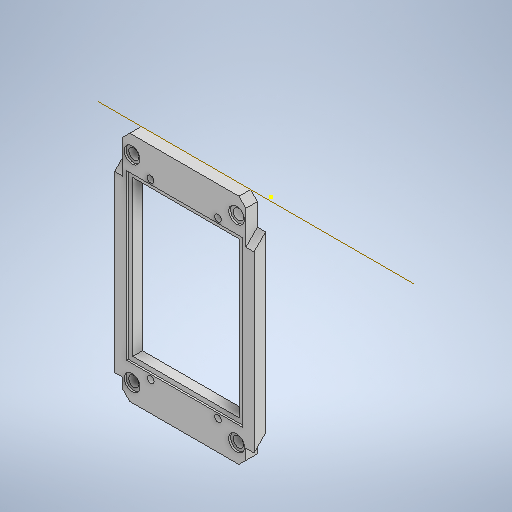
# Autodesk Inventor part: mirror_bracket
Saved by Autodesk Inventor 2025.1 (Build 291241000, 241)
## iProperties
Created: 2024-11-14
Part Number: mirror_bracket
Material: Ogólny
Document SubType Name: Modeling
Designer: PC
Density: 1 g/cm^3
Appearance: Domyślna
Author: PC
Autodesk Inventor part; units mm, degrees
ref_plane "YZ Plane" through (0, 0, 0) normal (1, 0, 0) x (0, 1, 0)
ref_plane "XZ Plane" through (0, 0, 0) normal (0, 1, 0) x (-1, 0, 0)
ref_plane "XY Plane" through (0, 0, 0) normal (0, 0, 1) x (1, 0, 0)
sketch "Szkic1" plane through (0, 0, 0) normal (0, 0, 1) x (1, 0, 0)
  circle A0 centre (-15, -14.1421) radius 2 projected
  circle A1 centre (-60, -14.1421) radius 2 projected
  circle A2 centre (-15, -98.9949) radius 2 projected
  circle A3 centre (-60, -98.9949) radius 2 projected
  line L0 (-75, -84.8528) -> (0, -84.8528) construction
  line L1 (-75, -27.2843) -> (0, -27.2843) construction
  line L2 (-12.5, -21.2132) -> (-62.5, -21.2132) construction
  line L3 (-62.5, -21.2132) -> (-62.5, -91.9239) construction
  line L4 (-62.5, -91.9239) -> (-12.5, -91.9239) construction
  line L5 (-12.5, -91.9239) -> (-12.5, -21.2132) construction
  line L6 (-15, -98.9949) -> (-60, -14.1421) construction
  line L7 (-15, -14.1421) -> (-60, -98.9949) construction
  line L8 (-7.5, -6.5685) -> (-67.5, -6.5685)
  line L9 (-67.5, -6.5685) -> (-67.5, -106.5685)
  line L10 (-67.5, -106.5685) -> (-7.5, -106.5685)
  line L11 (-7.5, -106.5685) -> (-7.5, -6.5685)
  circle A4 centre (-15, -14.1421) radius 2.25
  circle A5 centre (-60, -14.1421) radius 2.25
  circle A6 centre (-60, -98.9949) radius 2.25
  circle A7 centre (-15, -98.9949) radius 2.25
  line L12 (-12.5, -21.2132) -> (-62.5, -21.2132)
  line L13 (-62.5, -21.2132) -> (-62.5, -91.9239)
  line L14 (-62.5, -91.9239) -> (-12.5, -91.9239)
  line L15 (-12.5, -91.9239) -> (-12.5, -21.2132)
  line L16 (-14.5, -23.2132) -> (-60.5, -23.2132)
  line L17 (-60.5, -23.2132) -> (-60.5, -89.9239)
  line L18 (-60.5, -89.9239) -> (-14.5, -89.9239)
  line L19 (-14.5, -89.9239) -> (-14.5, -23.2132)
  ellipse E0 centre (-7.5, -14.1421) end of major axis (-7.5, -18.3848) minor radius 3 projected
  ellipse E1 centre (-67.5, -14.1421) end of major axis (-67.5, -18.3848) minor radius 3 projected
  ellipse E2 centre (-67.5, -98.9949) end of major axis (-67.5, -103.2376) minor radius 3 projected
  ellipse E3 centre (-7.5, -98.9949) end of major axis (-7.5, -103.2376) minor radius 3 projected
  line L20 (-11.5, -94.4949) -> (-11.5, -106.5685)
  line L21 (-11.5, -94.4949) -> (-7.5, -94.4949)
  line L22 (-37.5, -106.5685) -> (-37.5, -6.5685) construction
  line L23 (-63.5, -94.4949) -> (-63.5, -106.5685)
  line L24 (-63.5, -94.4949) -> (-67.5, -94.4949)
  line L25 (-7.5, -56.5685) -> (-67.5, -56.5685) construction
  line L26 (-11.5, -18.6421) -> (-11.5, -6.5685)
  line L27 (-11.5, -18.6421) -> (-7.5, -18.6421)
  line L28 (-63.5, -18.6421) -> (-63.5, -6.5685)
  line L29 (-63.5, -18.6421) -> (-67.5, -18.6421)
  point P0 (0, 0)
  point P1 (-37.5, -56.5685)
  point P2 (-37.5, -91.9239)
  point P3 (-12.5, -56.5685)
  point P4 (-37.5, -56.5685)
  dimension "d0" = 50
  dimension "d1" = 70.7107
  dimension "d2" = 4.5
  dimension "d3" = 2
  dimension "d4" = 60
  dimension "d5" = 100
  dimension "d15" = 4
  dimension "d16" = 4.5
  constraints: 56 end point, 9 symmetric about line, 8 midpoint, 8 parallel, 5 perpendicular, 4 centre point, 4 coincident, 4 horizontal, 3 equal radius, 2 horizontal alignment, 2 point on line, 2 vertical alignment, 1 vertical, 3 other
  measures "d0" distance of L3.end L4.end
  measures "d1" distance of L4.end L2.start
  measures "d2" diameter of A4
  measures "d3" distance between parallel lines of L15 L19
  measures "d4" distance of L9.end L10.end
  measures "d5" distance of L8.end L9.end
  measures "d15" distance from line of E3.centre L20
  measures "d16" distance from line of L21 E3.centre
extrude "Wyciągnięcie proste1" add sketch "Szkic1" along normal blind 5 contours L11 E0 L27 L26 L8 | L26 L27 L11 L21 L20 L10 L23 L24 L9 L29 L28 L8 | L11 E0 | L28 L29 L9 E1 L8 | E1 L9 | L11 E3 L10 L20 L21 | L24 L23 L10 L9 E2 | L11 E3 | E2 L9 | L15 L14 L13 L12 picked at (-8.4985, -14.0649) picked at (-66.5015, -14.2193) picked at (-8.4985, -98.9177) picked at (-66.5015, -99.0721)
sketch "Szkic2" plane through (0, 0, 5) normal (0, 0, 1) x (1, 0, 0)
  line L0 (-62.5, -21.2132) -> (-62.5, -91.9239) projected
  line L1 (-12.5, -21.2132) -> (-62.5, -21.2132) construction
  line L2 (-12.5, -91.9239) -> (-12.5, -21.2132) projected
  line L3 (-62.5, -91.9239) -> (-12.5, -91.9239) construction
  line L4 (-12.5, -21.2132) -> (-62.5, -21.2132)
  line L5 (-62.5, -21.2132) -> (-62.5, -91.9239)
  line L6 (-62.5, -91.9239) -> (-12.5, -91.9239)
  line L7 (-12.5, -91.9239) -> (-12.5, -21.2132)
  circle A0 centre (-15, -14.1421) radius 3.4
  circle A1 centre (-60, -14.1421) radius 3.4
  circle A2 centre (-60, -98.9949) radius 3.4
  circle A3 centre (-15, -98.9949) radius 3.4
  point P0 (0, 0)
  dimension "d10" = 6.8
  dimension "d11" = 6.8
  constraints: 8 end point, 4 centre point, 4 coincident, 2 equal radius, 2 parallel, 1 horizontal, 1 perpendicular
  measures "d10" diameter of A0
  measures "d11" diameter of A1
extrude "Wyciągnięcie proste2" cut sketch "Szkic2" against normal blind 0.8
chamfer "Faza1" distance 3 angle 45 4 edges at (-7.5, -106.5685, 2.5) (-67.5, -106.5685, 2.5) (-67.5, -6.5685, 2.5) (-7.5, -6.5685, 2.5)
sketch "Szkic3" plane through (0, 0, 5) normal (0, 0, 1) x (1, 0, 0)
  point P0 (0, 0)
ref_plane "Płaszczyzna konstrukcyjna1" through (-7.5, -6.5685, 0) normal (0, 0.7071, -0.7071) x (-1, 0, 0)
sketch "Szkic4" plane through (-7.5, -6.5685, 0) normal (0, 0.7071, -0.7071) x (-1, 0, 0)
  circle A0 centre (0, -65.3553) radius 3 projected
  circle A1 centre (0, -5.3553) radius 3 projected
  circle A2 centre (60, -65.3553) radius 3 projected
  circle A3 centre (60, -5.3553) radius 3 projected
  line L0 (0, -68.5894) -> (0, -2.1213) projected
  line L1 (57, -70.7107) -> (3, -70.7107) projected
  line L2 (3, 3.5355) -> (57, 3.5355) projected
  line L3 (0, -76.8553) -> (3.5, -76.8553)
  line L4 (3.5, -76.8553) -> (3.5, -61.8553)
  line L5 (3.5, -61.8553) -> (0, -61.8553)
  line L6 (0, -61.8553) -> (0, -76.8553)
  line L7 (0, -65.3553) -> (0, -5.3553) construction
  line L8 (0, -5.3553) -> (60, -5.3553) construction
  line L9 (0, -35.3553) -> (60, -35.3553) construction
  line L10 (60, -2.1213) -> (60, -68.5894) construction
  line L11 (30, -70.7107) -> (30, -5.3553) construction
  line L12 (0, 6.1447) -> (3.5, 6.1447)
  line L13 (3.5, 6.1447) -> (3.5, -8.8553)
  line L14 (3.5, -8.8553) -> (0, -8.8553)
  line L15 (0, -8.8553) -> (0, 6.1447)
  line L16 (60, -76.8553) -> (56.5, -76.8553)
  line L17 (56.5, -76.8553) -> (56.5, -61.8553)
  line L18 (56.5, -61.8553) -> (60, -61.8553)
  line L19 (60, -61.8553) -> (60, -76.8553)
  line L20 (56.5, 6.1447) -> (56.5, -8.8553)
  line L21 (60, 6.1447) -> (56.5, 6.1447)
  line L22 (60, -8.8553) -> (60, 6.1447)
  line L23 (56.5, -8.8553) -> (60, -8.8553)
  point P0 (-7.5, 4.6447)
  point P1 (56.5, -70.7107)
  point P2 (0, -8.3553)
  point P3 (0, -8.8553)
  point P4 (0, -2.1213)
  point P5 (0, -2.3553)
  point P6 (3.5, -70.7107)
  point P7 (0, -61.8553)
  point P8 (60, -68.3553)
  point P9 (60, -62.3553)
  point P10 (60, -8.3553)
  point P11 (60, -2.3553)
  point P12 (0, -62.3553)
  point P13 (0, -68.3553)
  dimension "d18" = 3.5
  dimension "d19" = 15
  dimension "d22" = 3.5
  constraints: 40 end point, 12 symmetric about line, 4 midpoint, 2 collinear, 2 parallel, 2 perpendicular, 1 horizontal
  measures "d18" distance of L4.end L5.end
  measures "d19" distance of L3.end L4.end
  measures "d22" distance from line of L5 L7.start
extrude "Wyciągnięcie proste3" cut sketch "Szkic4" against normal through all contours A0 L0 | A0 L0 L5 L4 L3 L6 | L20 L21 L22 A3 L23 | L0 A1 L15 L12 L13 L14 | L17 L18 L19 A2 L16 | L0 A1 | A1 L0 | A2 L19 | L22 A3 picked at (1.6278, -64.5387) picked at (59.5353, -64.4698) picked at (59.296, -4.4408)
chamfer "Faza2" distance 3 angle 45 4 edges at (-11, -6.5685, 2.5) (-64, -6.5685, 2.5) (-11, -106.5685, 2.5) (-64, -106.5685, 2.5)
sketch "Szkic5" plane through (0, 0, 5) normal (0, 0, 1) x (1, 0, 0)
  point P0 (0, 0)
sketch "Szkic6" plane through (0, 0, 5) normal (0, 0, 1) x (1, 0, 0)
  circle A0 centre (-52, -19.2132) radius 1.45
  line L0 (-14, -6.5685) -> (-61, -6.5685) construction
  line L1 (-37.5, -6.5685) -> (-37.5, -106.5685) construction
  line L2 (-61, -106.5685) -> (-14, -106.5685) construction
  line L3 (-67.5, -19.0919) -> (-67.5, -94.0452) construction
  line L4 (-67.5, -56.5685) -> (-7.5, -56.5685) construction
  line L5 (-7.5, -94.0452) -> (-7.5, -19.0919) construction
  line L6 (-62.5, -21.2132) -> (-12.5, -21.2132) construction
  line L7 (-64, -9.5685) -> (-64, -24.0919) construction
  circle A1 centre (-23, -19.2132) radius 1.45
  circle A2 centre (-52, -93.9239) radius 1.45
  circle A3 centre (-23, -93.9239) radius 1.45
  point P0 (0, 0)
  dimension "d26" = 2.9
  dimension "d27" = 2
  dimension "d28" = 12
  constraints: 4 centre point, 4 end point, 4 midpoint, 3 symmetric about line, 3 other
  measures "d26" diameter of A0
  measures "d27" distance from line of L6 A0.centre
  measures "d28" distance from line of L7 A0.centre
extrude "Wyciągnięcie proste4" cut sketch "Szkic6" against normal through all
